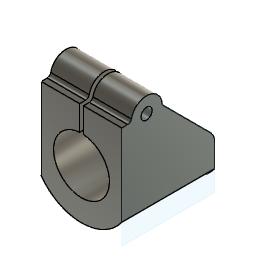
Pinch_Fit_Cap v3 (Autodesk Fusion 360 design; units mm, degrees)
Autodesk Fusion 360 part; units mm, degrees
note: some values were not read from the file. Set by a fixed rule: which sketch regions a step uses.
sketch "Sketch1" plane through (0, 0, 0) normal (1, 0, 0) x (0, 1, 0)
  line L0 (-70, 0) -> (110, 0)
  line L1 (0, 110) -> (0, -170)
  line L2 (-15.2069, 0) -> (-20, 0)
  line L3 (-20, 0) -> (-20, -82.5)
  line L4 (-20, -82.5) -> (55, -82.5)
  line L5 (55, -82.5) -> (55, -47.4706)
  line L6 (51.4853, -38.9853) -> (13.3243, -0.8243)
  line L7 (55, -42.5) -> (115.1063, -42.5) construction
  arc A0 (12.4562, 1.046) -> (-12.2636, 2.4194) centre (0, 0) ccw
  arc A1 (-15.2069, 0) -> (-12.2636, 2.4194) centre (-15.2069, 3) ccw
  arc A2 (12.4562, 1.046) -> (13.3243, -0.8243) centre (15.4456, 1.297) ccw
  arc A3 (55, -47.4706) -> (51.4853, -38.9853) centre (43, -47.4706) ccw
  point P0 (-12.5, 0)
  dimension "d2" = 7.5
  dimension "d3" = 82.5
  dimension "d4" = 75
  dimension "d5" = 40
  dimension "d6" = 135
  dimension "d7" = 12.5
  dimension "d8" = 3
  dimension "d9" = 3
  dimension "d10" = 12
  constraint coincident A0.centre origin
  constraint horizontal L0
  constraint vertical L1
  constraint coincident L0 P0
  constraint parallel L0 L2
  constraint perpendicular L2 L3
  constraint perpendicular L1 L4
  constraint perpendicular L4 L5
  constraint horizontal L7
  constraint coincident P0 L2
  constraint coincident P0 A0
  constraint tangent A0 A1
  constraint tangent L2 A1
  constraint tangent A0 A2
  constraint tangent L6 A2
  constraint coincident L7.start L6
  constraint coincident L7.start L5
  constraint tangent L6 A3
  constraint tangent L5 A3
  measures "d2" distance of P0 L2.end
  measures "d3" distance of L2.end L3.end
  measures "d4" distance of L3.end L4.end
  measures "d5" distance of L4.end L7.start
  measures "d6" angle of L6 L7
  measures "d7" radius of A0
  measures "d8" radius of A1
  measures "d9" radius of A2
  measures "d10" radius of A3
extrude "Extrude1" add sketch "Sketch1" along normal blind 65
sketch "Sketch2" plane through (65, 0, 0) normal (1, 0, 0) x (0, 1, 0)
  line L0 (-15.2069, 0) -> (-20, 0)
  line L1 (-20, 0) -> (-20, -82.5)
  line L2 (-20, -82.5) -> (55, -82.5)
  line L3 (55, -82.5) -> (55, -47.4706)
  arc A0 (55, -47.4706) -> (51.4853, -38.9853) centre (43, -47.4706) ccw
  line L4 (51.4853, -38.9853) -> (13.3243, -0.8243)
  arc A1 (12.4562, 1.046) -> (13.3243, -0.8243) centre (15.4456, 1.297) ccw
  arc A2 (12.4562, 1.046) -> (-12.2636, 2.4194) centre (0, 0) ccw
  arc A3 (-15.2069, 0) -> (-12.2636, 2.4194) centre (-15.2069, 3) ccw
sketch "Sketch3" plane through (0, -20, 0) normal (0, -1, 0) x (1, 0, 0)
  line L0 (0, 0) -> (0, -82.5)
  line L1 (0, -82.5) -> (65, -82.5)
  line L2 (65, -82.5) -> (65, 0)
  line L3 (65, 0) -> (0, 0)
  line L4 (0, 0) -> (32.5, 0)
  line L5 (32.5, 0) -> (32.5, -42.5)
  circle A0 centre (32.5, -42.5) radius 22.5
  dimension "d13" = 42.5
  dimension "d14" = 45
  constraint coincident L0.start L3.end
  constraint midpoint L3 L4.end
  constraint perpendicular L3 L5
  constraint coincident L5.end A0.centre
  measures "d13" distance of L4.end L5.end
  measures "d14" diameter of A0
extrude "Extrude2" cut sketch "Sketch3" against normal blind 110 contours A0
sketch "Sketch4" plane through (0, -20, 0) normal (0, -1, 0) x (1, 0, 0)
  circle A0 centre (32.5, -42.5) radius 22.5
  line L0 (0, 0) -> (0, -82.5)
  line L1 (0, -82.5) -> (65, -82.5)
  line L2 (65, -82.5) -> (65, 0)
  line L3 (65, 0) -> (0, 0)
  circle A1 centre (32.5, -42.5) radius 40
  dimension "d17" = 80
  constraint concentric A0 A1
  measures "d17" diameter of A1
extrude "Extrude3" cut sketch "Sketch4" against normal blind 110 contours L0 L1 A1 | L1 L2 A1
sketch "Sketch5" plane through (0, 0, 0) normal (0, 1, 0) x (1, 0, 0)
sketch "Sketch6" plane through (65, 0, 0) normal (1, 0, 0) x (0, 1, 0)
  circle A0 centre (0, 0) radius 4.5
  dimension "d23" = 9
  constraint coincident A0.centre origin
  measures "d23" diameter of A0
extrude "Extrude4" cut sketch "Sketch6" against normal blind 120
sketch "Sketch7" plane through (65, 17.5, -34.7081) normal (1, 0, 0) x (0, 1, 0)
sketch "Sketch8" plane through (0, 0, 0) normal (-1, 0, 0) x (0, -1, 0)
  circle A0 centre (0, 0) radius 4.5
  line L0 (-55, -65.8184) -> (20, -65.8184)
  line L1 (20, -65.8184) -> (20, 0)
  line L2 (20, 0) -> (15.2069, 0)
  arc A1 (12.2636, 2.4194) -> (15.2069, 0) centre (15.2069, 3) ccw
  arc A2 (12.2636, 2.4194) -> (-12.4562, 1.046) centre (0, 0) ccw
  arc A3 (-13.3243, -0.8243) -> (-12.4562, 1.046) centre (-15.4456, 1.297) ccw
  line L3 (-13.3243, -0.8243) -> (-51.4853, -38.9853)
  arc A4 (-51.4853, -38.9853) -> (-55, -47.4706) centre (-43, -47.4706) ccw
  line L4 (-55, -47.4706) -> (-55, -65.8184)
  circle A5 centre (0, 0) radius 7.5
  dimension "d26" = 15
  constraint concentric A0 A5
  measures "d26" diameter of A5
extrude "Extrude5" cut sketch "Sketch8" against normal blind 8 contours A5
sketch "Sketch9" plane through (0, -20, 0) normal (0, -1, 0) x (1, 0, 0)
  circle A0 centre (32.5, -42.5) radius 22.5
  arc A1 (0, -65.8184) -> (65, -65.8184) centre (32.5, -42.5) ccw
  line L0 (65, -65.8184) -> (65, 0)
  line L1 (65, 0) -> (0, 0)
  line L2 (0, 0) -> (0, -65.8184)
  line L3 (31, -42.5) -> (34, -42.5)
  line L4 (34, -42.5) -> (34, 31.8842)
  line L5 (34, 31.8842) -> (31, 31.8842)
  line L6 (31, 31.8842) -> (31, -42.5)
  dimension "d30" = 3
  constraint horizontal L3
  constraint vertical L4
  constraint horizontal L5
  constraint vertical L6
  measures "d30" distance of L4 L6
extrude "Extrude6" cut sketch "Sketch9" against normal blind 130 contours A0 L3 L4 L6 | A0 L1 L4 L6 | L1 L4 L5 L6 picked at (31.959, -57.4579)
